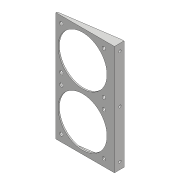
# Autodesk Inventor part: Fan_Bracket
Saved by Autodesk Inventor 2018 (Build 220112000, 112)
## iProperties
Created: 2019-09-19
Part Number: Fan_Bracket
Material: Generic
Document SubType Name: Modeling
Designer: Clevo
Density: 1 g/cm^3
Appearance: Default
Author: Clevo
Autodesk Inventor part; units mm, degrees
ref_plane "YZ Plane" through (0, 0, 0) normal (1, 0, 0) x (0, 1, 0)
ref_plane "XZ Plane" through (0, 0, 0) normal (0, 1, 0) x (-1, 0, 0)
ref_plane "XY Plane" through (0, 0, 0) normal (0, 0, 1) x (1, 0, 0)
sketch "Sketch1" plane through (0, 0, 0) normal (0, 1, 0) x (-1, 0, 0)
  line L0 (-26.5, -50) -> (26.5, -50)
  line L1 (26.5, -50) -> (26.5, 50)
  line L2 (26.5, 50) -> (-26.5, 50)
  line L3 (-26.5, 50) -> (-26.5, -50)
  line L4 (-26.5, -50) -> (26.5, 50) construction
  line L5 (26.5, -50) -> (-26.5, 50) construction
  point P0 (0, 0)
  dimension "d0" = 53
  dimension "d1" = 100
  constraints: 12 end point, 2 midpoint, 2 parallel, 1 horizontal, 1 perpendicular
  measures "d0" distance of L1.end L2.end
  measures "d1" distance of L0.end L1.end
extrude "Extrusion1" add sketch "Sketch1" along normal blind 1.2
sketch "Sketch2" plane through (26.5, 0, 50) normal (1, 0, 0) x (0, 0, -1)
  line L0 (100, 0) -> (0, 0) projected
  line L1 (0, 0) -> (100, 0)
  line L2 (100, 0) -> (100, 9)
  line L3 (100, 9) -> (0, 9)
  line L4 (0, 9) -> (0, 0)
  point P0 (50, 0)
  dimension "d4" = 9
  constraints: 8 end point, 2 parallel, 1 horizontal, 1 perpendicular
  measures "d4" distance of L1.end L2.end
extrude "Extrusion2" add sketch "Sketch2" along normal blind 2
sketch "Sketch3" plane through (26.5, 1.2, 50) normal (0, 0, 1) x (1, 0, 0)
  line L0 (-53, -1.2) -> (2, -1.2) projected
  line L1 (2, 7.8) -> (2, -1.2) projected
  line L2 (0, 7.8) -> (2, 7.8) projected
  line L3 (0, 7.8) -> (0, 0) projected
  line L4 (-53, 0) -> (0, 0) projected
  line L5 (-53, -1.2) -> (-53, 0) projected
  line L6 (0, 7.8) -> (2, 7.8) projected
  line L7 (-53, 0) -> (0, 7.8)
  point P0 (-26.5, -1.2)
  constraints: 2 end point
extrude "Extrusion3" add sketch "Sketch3" along normal blind 1.5
mirror "Mirror1" about plane through (0, 0, 0) normal (0, 0, 1) of "Extrusion3"
sketch "Sketch4" plane through (26.5, 0, 50) normal (-1, 0, 0) x (0, 0, 1)
  line L0 (0, 1.2) -> (-100, 1.2) projected
  line L1 (0, 9) -> (0, 1.2) projected
  line L2 (-100, 9) -> (0, 9) projected
  line L3 (-100, 1.2) -> (-100, 9) projected
  line L4 (-5, 5.1) -> (-95, 5.1)
  line L5 (-100, 1.2) -> (0, 1.2) projected
  point P0 (-50, 0)
  point P1 (0, 5.1)
  point P2 (-50, 5.1)
  point P3 (-50, 9)
  dimension "d9" = 90
  constraints: 3 midpoint, 2 end point, 1 horizontal alignment, 1 parallel, 1 vertical alignment
  measures "d9" distance of L4.start L4.end
hole "Hole1" at (26.5, 5.1, 45) at (26.5, 5.1, 0) at (26.5, 5.1, -45) direction (1, 0, 0) diameter 2.4 end through all clearance for "Flat Head Machine Screw" size "M2" standard "Ansi Metric M Profile"
sketch "Sketch5" plane through (0, 1.2, 0) normal (0, 1, 0) x (1, 0, 0)
  circle A0 centre (-1.5, -25) radius 23
  line L0 (18.5, -5) -> (-21.5, -5)
  line L1 (-21.5, -5) -> (-21.5, -45)
  line L2 (-21.5, -45) -> (18.5, -45)
  line L3 (18.5, -45) -> (18.5, -5)
  line L4 (18.5, -5) -> (-21.5, -45) construction
  line L5 (-21.5, -5) -> (18.5, -45) construction
  line L6 (-26.5, 50) -> (-26.5, -50) projected
  point P0 (0, 0)
  dimension "d17" = 46
  dimension "d18" = 40
  dimension "d19" = 40
  dimension "d20" = 25
  dimension "d21" = 25
  constraints: 12 end point, 2 midpoint, 2 parallel, 1 centre point, 1 horizontal, 1 perpendicular
  measures "d17" diameter of A0
  measures "d18" distance of L0.end L1.end
  measures "d19" distance of L1.end L2.end
  measures "d20" vertical distance of A0.centre point (0, 0)
  measures "d21" distance from line of L6 A0.centre
extrude "Extrusion4" cut sketch "Sketch5" against normal through all contours A0 L3 | L3 A0 L2 L1 L0 | L0 A0 | A0 L2 | L1 A0
hole "Hole2" at (-21.5, 1.2, 45) at (-21.5, 1.2, 5) at (18.5, 1.2, 5) at (18.5, 1.2, 45) direction (0, -1, 0) diameter 3.2 end through all clearance for "Flat Head Machine Screw" size "M3" standard "Ansi Metric M Profile"
mirror "Mirror2" about plane through (0, 0, 0) normal (0, 0, 1) of "Hole2", "Extrusion4"
equation "\"d19\" = d18"
body "Solid1"
